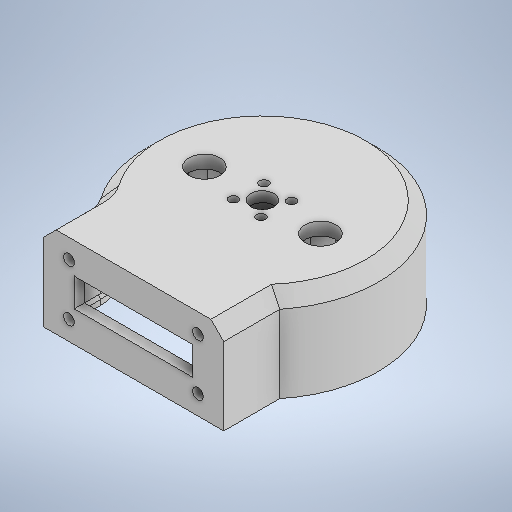
# Autodesk Inventor part: SCARA arm base
Saved by Autodesk Inventor 2025.2 (Build 292293000, 293)
## iProperties
Created: 2025-01-26
Part Number: SCARA arm base
Material: Generic
Document SubType Name: Modeling
Designer: caomi
Density: 1 g/cm^3
Appearance: Default
Author: caomi
Autodesk Inventor part; units mm, degrees
ref_plane "YZ Plane" through (0, 0, 0) normal (1, 0, 0) x (0, 1, 0)
ref_plane "XZ Plane" through (0, 0, 0) normal (0, 1, 0) x (-1, 0, 0)
ref_plane "XY Plane" through (0, 0, 0) normal (0, 0, 1) x (1, 0, 0)
sketch "Sketch1" plane through (0, 0, 0) normal (0, 1, 0) x (-1, 0, 0)
  circle A0 centre (0, 0) radius 45
  line L0 (89.3923, 0) -> (-44.3923, 0) construction
  line L1 (33.5, 5) -> (33.5, -5)
  line L2 (33.5, -5) -> (29.5, -8.3)
  line L3 (29.5, -8.3) -> (29.5, -15.35)
  line L4 (29.5, -15.35) -> (19.5, -15.35)
  line L5 (19.5, -15.35) -> (17.5, -17)
  line L6 (17.5, -17) -> (11.5, -17)
  line L7 (11.5, 17) -> (17.5, 17)
  line L8 (17.5, 17) -> (19.5, 15.35)
  line L9 (19.5, 15.35) -> (29.5, 15.35)
  line L10 (29.5, 15.35) -> (29.5, 8.3)
  line L11 (29.5, 8.3) -> (33.5, 5)
  line L12 (11.5, -17) -> (11.5, -7.25)
  line L13 (11.5, -7.25) -> (12.5, -6.25)
  line L14 (12.5, -6.25) -> (12.5, 6.25)
  line L15 (12.5, 6.25) -> (11.5, 7.25)
  line L16 (11.5, 7.25) -> (11.5, 17)
  circle A1 centre (22.5, 0) radius 6
  line L17 (13.233, 0) -> (-58.233, 0) construction
  line L18 (-33.5, -5) -> (-33.5, 5)
  line L19 (-33.5, 5) -> (-29.5, 8.3)
  line L20 (-29.5, 8.3) -> (-29.5, 15.35)
  line L21 (-29.5, 15.35) -> (-19.5, 15.35)
  line L22 (-19.5, 15.35) -> (-17.5, 17)
  line L23 (-17.5, 17) -> (-11.5, 17)
  line L24 (-11.5, -17) -> (-17.5, -17)
  line L25 (-17.5, -17) -> (-19.5, -15.35)
  line L26 (-19.5, -15.35) -> (-29.5, -15.35)
  line L27 (-29.5, -15.35) -> (-29.5, -8.3)
  line L28 (-29.5, -8.3) -> (-33.5, -5)
  line L29 (-11.5, 17) -> (-11.5, 7.25)
  line L30 (-11.5, 7.25) -> (-12.5, 6.25)
  line L31 (-12.5, 6.25) -> (-12.5, -6.25)
  line L32 (-12.5, -6.25) -> (-11.5, -7.25)
  line L33 (-11.5, -7.25) -> (-11.5, -17)
  circle A2 centre (-22.5, 0) radius 6
  line L34 (0, -29.964) -> (0, 34.746) construction
  line L35 (-35, 28.2843) -> (-35, 50)
  line L36 (-35, 50) -> (35, 50)
  line L37 (35, 50) -> (35, 28.2843)
  line L38 (-29.6, 8.3471) -> (-33.6, 5.0471)
  line L39 (-33.6, 5.0471) -> (-33.6, -5.0471)
  line L40 (-33.6, -5.0471) -> (-29.6, -8.3471)
  line L41 (-29.6, -8.3471) -> (-29.6, -15.45)
  line L42 (-29.6, -15.45) -> (-19.5359, -15.45)
  line L43 (-19.5359, -15.45) -> (-17.5359, -17.1)
  line L44 (-17.5359, -17.1) -> (-11.4, -17.1)
  line L45 (-11.4, -17.1) -> (-11.4, -7.2086)
  line L46 (-11.4, -7.2086) -> (-12.4, -6.2086)
  line L47 (-12.4, -6.2086) -> (-12.4, 6.2086)
  line L48 (-12.4, 6.2086) -> (-11.4, 7.2086)
  line L49 (-11.4, 7.2086) -> (-11.4, 17.1)
  line L50 (-11.4, 17.1) -> (-17.5359, 17.1)
  line L51 (-17.5359, 17.1) -> (-19.5359, 15.45)
  line L52 (-19.5359, 15.45) -> (-29.6, 15.45)
  line L53 (-29.6, 15.45) -> (-29.6, 8.3471)
  line L54 (11.4, 17.1) -> (17.5359, 17.1)
  line L55 (17.5359, 17.1) -> (19.5359, 15.45)
  line L56 (19.5359, 15.45) -> (29.6, 15.45)
  line L57 (29.6, 15.45) -> (29.6, 8.3471)
  line L58 (29.6, 8.3471) -> (33.6, 5.0471)
  line L59 (33.6, 5.0471) -> (33.6, -5.0471)
  line L60 (33.6, -5.0471) -> (29.6, -8.3471)
  line L61 (29.6, -8.3471) -> (29.6, -15.45)
  line L62 (29.6, -15.45) -> (19.5359, -15.45)
  line L63 (19.5359, -15.45) -> (17.5359, -17.1)
  line L64 (17.5359, -17.1) -> (11.4, -17.1)
  line L65 (11.4, -17.1) -> (11.4, -7.2086)
  line L66 (11.4, -7.2086) -> (12.4, -6.2086)
  line L67 (12.4, -6.2086) -> (12.4, 6.2086)
  line L68 (12.4, 6.2086) -> (11.4, 7.2086)
  line L69 (11.4, 7.2086) -> (11.4, 17.1)
  point P0 (11.5, -12.125)
  point P1 (-11.5, 12.125)
  dimension "d0" = 45
  dimension "d2" = 34
  dimension "d3" = 6
  dimension "d4" = 8
  dimension "d5" = 11
  dimension "d6" = 12
  dimension "d7" = 18
  dimension "d8" = 16.6
  dimension "d9" = 12.5
  dimension "d10" = 1
  dimension "d11" = 10
  dimension "d13" = 22
  dimension "d16" = 8
  dimension "d17" = 11
  dimension "d19" = 18
  dimension "d20" = 16.6
  dimension "d22" = 1
  dimension "d24" = 45
  dimension "d25" = 22
  dimension "d26" = 34
  dimension "d27" = 45
  dimension "d28" = 90
  dimension "d48" = 70
  dimension "d49" = 50
  dimension "d91" = 0.1
  dimension "d92" = 0.1
  constraints: 140 end point, 23 parallel, 10 perpendicular, 6 midpoint, 5 point on line, 4 collinear, 4 vertical, 3 centre point, 2 horizontal, 2 point on circle, 1 coincident, 1 equal radius, 46 other
  measures "d0" angle of L12 L13
  measures "d2" distance between parallel lines of L7 L6
  measures "d3" distance of L5.end L12.start
  measures "d4" distance from line of L12 L4.end
  measures "d5" distance from line of A1.centre L16
  measures "d6" diameter of A1
  measures "d7" distance between parallel lines of L12 L3
  measures "d8" distance of L2.end L11.start
  measures "d9" distance of L14.start L14.end
  measures "d10" distance between parallel lines of L14 L12
  measures "d11" distance of L1.start L1.end
  measures "d13" distance from line of point (-11.5, 12.125) L18
  measures "d16" distance from line of L29 L21.end
  measures "d17" distance from line of A2.centre L33
  measures "d19" distance between parallel lines of L29 L20
  measures "d20" distance of L19.end L28.start
  measures "d22" distance between parallel lines of L31 L29
  measures "d24" angle of L30 L29
  measures "d25" distance between parallel lines of L12 L1
  measures "d26" distance between parallel lines of L23 L24
  measures "d27" distance of A2.centre A1.centre
  measures "d28" diameter of A0
  measures "d48" distance of L35.end L36.end
  measures "d49" distance from line of L36 point (0, 0)
  measures "d91" distance between parallel lines of L20 L53
  measures "d92" distance between parallel lines of L16 L69
extrude "Extrusion1" add sketch "Sketch1" against normal blind 30 contours A0 | A0 L35 L36 L37
extrude "Extrusion2" add sketch "Sketch1" along normal blind 5 contours A0 | A0 L35 L36 L37 | L1 L2 L3 L4 L5 L6 L12 L13 L14 L15 L16 L7 L8 L9 L10 L11 | L18 L19 L20 L21 L22 L23 L29 L30 L31 L32 L33 L24 L25 L26 L27 L28 | L53 L52 L51 L50 L49 L48 L47 L46 L45 L44 L43 L42 L41 L40 L39 L38 | L54 L55 L56 L57 L58 L59 L60 L61 L62 L63 L64 L65 L66 L67 L68 L69
fillet "Fillet1" radius 10 1 edges at (-35, -12.5, 28.2843)
chamfer "Chamfer1" distance 5 angle 45 4 edges at (35, 5, 39.1421) (1.5099, 5, -44.9747) (-35.4654, 5, 28.6077) (-35, 5, 40.8114)
shell "Shell2" thickness 4 removed faces 1 at (3.8, -30, 39.0333)
sketch "Sketch2" plane through (0, 1, 0) normal (0, -1, 0) x (-0.9987274, 0, -0.0504346)
  circle A0 centre (-5.6569, -5.6569) radius 1.75
  circle A1 centre (0, 0) radius 5
  circle A2 centre (0, 0) radius 4.5
  line L0 (-5.6569, -5.6569) -> (0, 0) construction
  line L1 (0, 0) -> (-7.2952, 0) construction
  circle A3 centre (0, 0) radius 11.25
  dimension "d35" = 3.5
  dimension "d36" = 8
  dimension "d42" = 10
  dimension "d50" = 45
  dimension "d73" = 22.5
  dimension "d93" = 9
  constraints: 4 centre point, 4 end point, 3 coincident, 1 horizontal
  measures "d35" diameter of A0
  measures "d36" distance of point (0, 0) L0.start
  measures "d42" diameter of A1
  measures "d50" angle of L0 L1
  measures "d73" diameter of A3
  measures "d93" diameter of A2
extrude "Extrusion9" cut sketch "Sketch2" along normal up to surface (31 mm away) contours A3
extrude "Extrusion10" add sketch "Sketch2" along normal blind 9.5 contours A0 | A3
extrude "Extrusion3" cut sketch "Sketch2" along normal through all both and the other way through all contours A0
pattern_circular "Circular Pattern1" count 4 over 360 about axis through (0, 0, 0) along (0, -1, 0) of "Extrusion3"
extrude "Extrusion11" cut sketch "Sketch2" against normal through all contours A2
ref_plane "Work Plane2" through (0, -27, 0) normal (0, -1, 0) x (1, 0, 0)
sketch "Sketch5" plane through (0, -27, 0) normal (0, -1, 0) x (1, 0, 0)
  line L0 (31, 46) -> (31, 26.8328) projected
  arc A0 (31, 31.6228) -> (33.5455, 23.5733) centre (45, 31.6228) ccw projected
  arc A1 (-33.5455, 23.5733) -> (31, 26.8328) centre (0, 0) ccw projected
  arc A2 (-33.5455, 23.5733) -> (-31, 31.6228) centre (-45, 31.6228) ccw projected
  line L1 (-31, 31.6228) -> (-31, 46) projected
ref_plane "Work Plane3" through (31, -27, 46) normal (0, 0, -1) x (-1, 0, 0)
sketch "Sketch6" plane through (31, -27, 46) normal (0, 0, -1) x (-1, 0, 0)
  line L0 (0, -1) -> (-1, 0)
  line L1 (-1, 0) -> (0, 1)
  line L2 (0, 25.3431) -> (0, -3) projected
  line L3 (0, -1) -> (0, 1)
  line L4 (-1, 0) -> (1.6557, 0) construction
  line L5 (0, -1) -> (0, 1)
  line L6 (94, 0) -> (-32, 0) projected
  point P0 (31, 27)
  point P1 (0, 28)
  point P2 (0, 0)
  point P3 (0, -1)
  point P4 (0, 1)
  dimension "d81" = 45
  dimension "d82" = 1
  constraints: 10 end point, 2 vertical, 1 collinear, 1 horizontal, 1 midpoint, 1 point on line, 1 other
  measures "d81" angle of L4 L1
  measures "d82" distance of L0.end point (0, 0)
sweep "Sweep1" cut profiles "Sketch6" path "Sketch5" path curves L0 A1 A2 L1
sketch "Sketch7" plane through (-35, -30, 50) normal (0, 0, 1) x (1, 0, 0)
  line L0 (0, 0) -> (0, 30) projected
  line L1 (70, 0) -> (0, 0) projected
  line L2 (5, 35) -> (65, 35) projected
  line L3 (58, 23) -> (58, 12)
  line L4 (58, 12) -> (12, 12)
  line L5 (12, 12) -> (12, 23)
  line L6 (12, 23) -> (58, 23)
  circle A0 centre (60, 27.5) radius 2.1
  circle A1 centre (60, 7.5) radius 2.1
  circle A2 centre (10, 7.5) radius 2.1
  circle A3 centre (10, 27.5) radius 2.1
  line L7 (60.6238, 17.5) -> (7.5466, 17.5) construction
  line L8 (35, -13.7005) -> (35, 51.7796) construction
  line L9 (70, 30) -> (70, 0) projected
  line L10 (0, 30) -> (5, 35) projected
  line L11 (65, 35) -> (70, 30) projected
  point P0 (35, 12)
  point P1 (58, 17.5)
  dimension "d85" = 12
  dimension "d86" = 20
  dimension "d87" = 50
  dimension "d88" = 4.2
  constraints: 12 end point, 4 centre point, 2 midpoint, 2 point on line, 1 horizontal, 1 vertical, 5 other
  measures "d85" distance between parallel lines of L1 L4
  measures "d86" distance of A1.centre A0.centre
  measures "d87" distance of A3.centre A0.centre
  measures "d88" diameter of A0
extrude "Extrusion12" cut sketch "Sketch7" against normal blind 20 contours L3 L4 L5 L6 | A0 | A1 | A2 | A3
equation "\"d17\" = d5"
body "Solid1"
